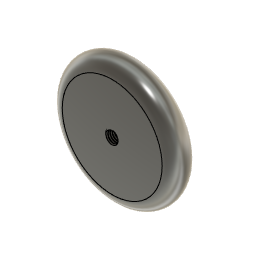
rotator wheel v3 (Autodesk Fusion 360 design; units mm, degrees)
Autodesk Fusion 360 part; units mm, degrees
sketch "outline" plane through (0, 0, 0) normal (0, 0, 1) x (1, 0, 0)
  line L0 (0, 0) -> (30, 0)
  arc A0 (30, 0) -> (30, 15) centre (30, 7.5) ccw
  line L1 (30, 15) -> (8, 19)
  line L2 (8, 19) -> (0, 19)
  line L3 (0, 19) -> (0, 0)
  dimension "d1" = 30
  dimension "d2" = 15
  dimension "d3" = 19
  dimension "d4" = 8
  dimension "d5" = 7.5
  constraint coincident L0.start L3.end
  constraint horizontal L0
  constraint tangent L0 A0
  constraint horizontal L2
  constraint perpendicular L0 L3
  measures "d1" distance of L0.start L0.end
  measures "d2" distance of L0.end A0.end
  measures "d3" distance of L0.start L2.end
  measures "d4" distance of L1.end L2.end
  measures "d5" radius of A0
revolve "Revolve1" add sketch "outline" angle 360 about axis through (0, 19, 0) along (0, -1, 0)
hole "Hole1" at (0, 19, 0) direction (0, -1, 0) diameter 6.78 end through all
thread "Thread1" "ISO Metric profile 8.0 M8x1.25 6H" major diameter 8.17 minor diameter 6.7795 pitch 1.25 angle 60 modelled right hand crest width 0.343 on face at (0.169, 12.6667, 3.3858) crest through (0, 18.6875, 3.3898)
named bodies: "rotator wheel"
